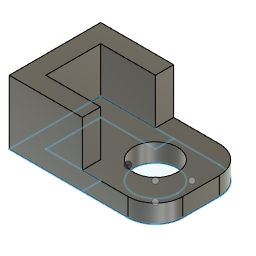
ex48 (Autodesk Fusion 360 design; units mm, degrees)
Autodesk Fusion 360 part; units mm, degrees
sketch "Sketch1" plane through (0, 0, 0) normal (0, 0, 1) x (1, 0, 0)
  line L0 (25, -25) -> (-40, -25)
  line L1 (-40, -25) -> (-40, 25)
  line L2 (-40, 25) -> (25, 25)
  line L3 (40, 10) -> (40, -10)
  arc A0 (40, 10) -> (25, 25) centre (25, 10) ccw
  arc A1 (25, -25) -> (40, -10) centre (25, -10) ccw
  line L4 (0, 15) -> (-30, 15)
  line L5 (0, -15) -> (-30, -15)
  line L6 (-30, 0) -> (-30, 15)
  line L7 (-30, 0) -> (-30, -15)
  line L8 (0, -15) -> (0, -25)
  circle A2 centre (15, 0) radius 12
  line L9 (0, 15) -> (0, 25)
  dimension "d2" = 50
  dimension "d3" = 15
  dimension "d4" = 15
  dimension "d8" = 15
  dimension "d9" = 24
  constraint horizontal L0
  constraint perpendicular L0 L1
  constraint parallel L0 L2
  constraint parallel L1 L3
  constraint tangent L3 A0
  constraint tangent L2 A0
  constraint tangent L3 A1
  constraint tangent L0 A1
  constraint perpendicular L2 L6
  constraint perpendicular L0 L7
  constraint coincident L0 L8.end
  constraint perpendicular L0 L8
  constraint coincident L2 L9.end
  constraint perpendicular L2 L9
  measures "d2" distance of L0.end L1.end
  measures "d3" radius of A0
  measures "d4" radius of A1
  measures "d8" distance of origin A2.centre
  measures "d9" diameter of A2
extrude "Extrude1" add sketch "Sketch1" along normal blind 35 contours L0 L1 L2 L4 L5 L6 L7 L8 L9
extrude "Extrude2" add sketch "Sketch1" along normal blind 10 contours L0 L2 L3 A0 A1 L4 L5 L6 L7 L8 L9
